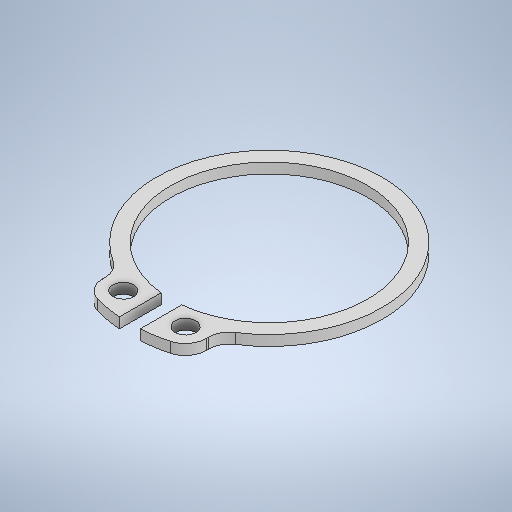
# Autodesk Inventor part: 49-01-001
Saved by Autodesk Inventor 2025.2 (Build 292293000, 293)
## iProperties
Created: 2024-11-28
Part Number: 49-01-001
Material: Generic
Document SubType Name: Modeling
Designer: Zvonko.Gabric
Density: 1 g/cm^3
Appearance: Default
Author: Zvonko.Gabric
Autodesk Inventor part; units mm, degrees
ref_plane "YZ Plane" through (0, 0, 0) normal (1, 0, 0) x (0, 1, 0)
ref_plane "XZ Plane" through (0, 0, 0) normal (0, 1, 0) x (-1, 0, 0)
ref_plane "XY Plane" through (0, 0, 0) normal (0, 0, 1) x (1, 0, 0)
sketch "Sketch1" plane through (0, 0, 0) normal (0, 1, 0) x (-1, 0, 0)
  line L0 (5.7554, 22.0444) -> (5.7554, 21.7775)
  line L1 (9.7554, 20.3898) -> (9.7554, 24.4055)
  circle A0 centre (7.7554, 22.0308) radius 1
  arc A1 (9.7554, 20.3898) -> (10.7554, 1.4426) centre (10.7554, 10.9426) ccw
  arc A2 (4.8407, 20.0976) -> (10.7554, 0.0432) centre (10.7554, 10.9426) ccw
  arc A3 (4.8407, 20.0976) -> (5.7554, 21.7775) centre (3.7554, 21.7775) ccw
  arc A4 (7.2337, 23.9751) -> (5.7554, 22.0444) centre (7.7554, 22.0444) ccw
  arc A5 (9.7554, 24.4055) -> (7.2337, 23.9751) centre (10.7554, 10.9426) ccw
  line L2 (10.7554, 25.4285) -> (10.7554, -6.744) construction
  line L3 (15.7554, 22.0444) -> (15.7554, 21.7775)
  line L4 (11.7554, 20.3898) -> (11.7554, 24.4055)
  circle A6 centre (13.7554, 22.0308) radius 1
  arc A7 (10.7554, 1.4426) -> (11.7554, 20.3898) centre (10.7554, 10.9426) ccw
  arc A8 (10.7554, 0.0432) -> (16.6701, 20.0976) centre (10.7554, 10.9426) ccw
  arc A9 (15.7554, 21.7775) -> (16.6701, 20.0976) centre (17.7554, 21.7775) ccw
  arc A10 (15.7554, 22.0444) -> (14.2772, 23.9751) centre (13.7554, 22.0444) ccw
  arc A11 (14.2772, 23.9751) -> (11.7554, 24.4055) centre (10.7554, 10.9426) ccw
  point P0 (0, 0)
  point P1 (9.7554, 22.3977)
  point P2 (11.7554, 22.3977)
  dimension "d0" = 2
  dimension "d1" = 2
  dimension "d2" = 13.5
  dimension "d3" = 9.5
  dimension "d4" = 10.8994
  dimension "d5" = 6
  dimension "d6" = 2
  constraints: 20 point on circle, 12 centre point, 10 end point, 9 symmetric about line, 2 midpoint, 2 point on line, 1 vertical, 6 other
  measures "d0" distance of point (9.755, 22.398) point (11.755, 22.398)
  measures "d1" diameter of A0
  measures "d2" radius of A5
  measures "d3" radius of A1
  measures "d4" radius of A2
  measures "d5" distance of A0.centre A6.centre
  measures "d6" radius of A3
extrude "Extrusion1" add sketch "Sketch1" along normal blind 1
body "Solid1"
